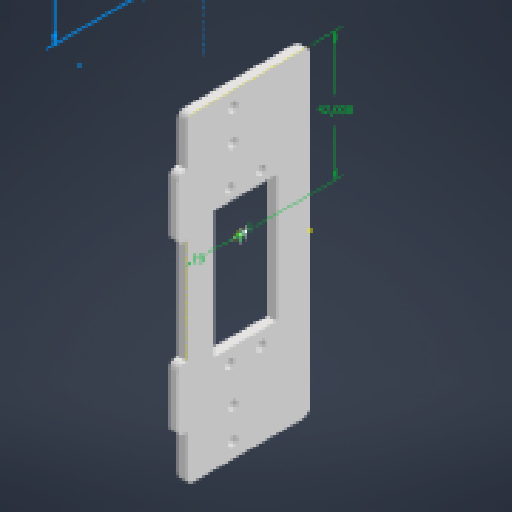
# Autodesk Inventor part: ParedEnsambleMotor
Saved by Autodesk Inventor 2026.2 (Build 302298010, 298A)
## iProperties
Created: 2026-04-28
Part Number: ParedEnsambleMotor
Material: Genérico
Document SubType Name: Modeling
Designer: Jose Carlos
Density: 1 g/cm^3
Appearance: Valor por defecto
Author: Jose Carlos
Autodesk Inventor part; units mm, degrees
ref_plane "YZ Plane" through (0, 0, 0) normal (1, 0, 0) x (0, 1, 0)
ref_plane "XZ Plane" through (0, 0, 0) normal (0, 1, 0) x (-1, 0, 0)
ref_plane "XY Plane" through (0, 0, 0) normal (0, 0, 1) x (1, 0, 0)
sketch "Boceto1" plane through (0, 0, 0) normal (1, 0, 0) x (0, 1, 0)
  line L0 (0, 0) -> (-52.0696, 0)
  line L1 (-52.0696, 0) -> (-52.0696, 40)
  line L2 (-52.0696, 40) -> (0, 40)
  line L3 (0, 40) -> (0, 0)
  line L4 (0, 0) -> (51.9461, 0)
  line L5 (51.9461, 0) -> (51.9461, 40)
  line L6 (51.9461, 40) -> (0, 40)
  line L7 (0, 40) -> (0, 0)
  line L8 (-52.0696, 43) -> (-52.0696, 40) construction
  line L9 (51.9461, 43) -> (51.9461, 40) construction
  line L10 (36.9461, 40) -> (16.9461, 40)
  line L11 (16.9461, 40) -> (16.9461, 43)
  line L12 (16.9461, 43) -> (36.9461, 43)
  line L13 (36.9461, 43) -> (36.9461, 40)
  line L14 (-17.0696, 40) -> (-37.0696, 40)
  line L15 (-37.0696, 40) -> (-37.0696, 43)
  line L16 (-37.0696, 43) -> (-17.0696, 43)
  line L17 (-17.0696, 43) -> (-17.0696, 40)
  point P0 (16.9461, 40)
  dimension "d15" = 40
  dimension "d16" = 20
  dimension "d17" = 3
  dimension "d18" = 15
  dimension "d19" = 3
  dimension "d20" = 20
  dimension "d21" = 15
  constraints: 32 end point, 8 parallel, 5 point on line, 4 horizontal, 4 perpendicular
  measures "d15" distance of L4.end L5.end
  measures "d16" distance of L11.end L12.end
  measures "d17" distance of L10.end L11.end
  measures "d18" distance between parallel lines of L5 L13
  measures "d19" distance of L14.end L15.end
  measures "d20" distance of L15.end L16.end
  measures "d21" distance between parallel lines of L1 L15
extrude "Extrusión1" add sketch "Boceto1" along normal blind 3
sketch "Boceto4" plane through (0, 0, 0) normal (-1, 0, 0) x (0, 0, 1)
  circle A0 centre (25, -37.0696) radius 1.6 construction
  circle A1 centre (25, -47.0696) radius 1.6 construction
  circle A2 centre (25, 36.9461) radius 1.6 construction
  circle A3 centre (25, 46.9461) radius 1.6 construction
  point P0 (0, 0)
hole "Agujero2" at (0, -47.0696, 25) at (0, -37.0696, 25) at (0, 36.9461, 25) at (0, 46.9461, 25) direction (1, 0, 0) diameter 3 end through all
sketch "Boceto5" plane through (3, 0, 0) normal (1, 0, 0) x (0, 0, -1)
  circle A0 centre (-23, 9.9416) radius 1.45 construction
  point P0 (0, 0)
hole "Agujero3" [suppressed]
sketch "ReferenciaEje" plane through (3, 0, 0) normal (1, 0, 0) x (0, 0, -1)
  circle A0 centre (-23, 9.9385) radius 1.65 construction
  line L0 (-40, 16.9461) -> (-40, -17.0696) construction
  line L1 (0, 51.9461) -> (-40, 51.9461) construction
  circle A1 centre (-21, 9.9385) radius 0.5
  point P0 (0, 0)
  dimension "d59" = 19
  dimension "d60" = 42.0076
  dimension "d61" = 1
  constraints: 2 coincident, 1 centre point
  measures "d59" distance from line of L0 point (-21, 9.938)
  measures "d60" distance from line of L1 point (-21, 9.938)
  measures "d61" diameter of A1
sketch "Boceto9" plane through (3, 0, 0) normal (1, 0, 0) x (0, 0, -1)
  circle A0 centre (-15.9, 24.6885) radius 2.25 construction
  circle A1 centre (-26.1, 24.6885) radius 2.25 construction
  circle A2 centre (-15.9, -24.8115) radius 2.25 construction
  circle A3 centre (-26.1, -24.8115) radius 2.25 construction
  point P0 (0, 0)
hole "Agujero4" at (3, 24.6885, 15.9) at (3, 24.6885, 26.1) at (3, -24.8115, 26.1) at (3, -24.8115, 15.9) direction (-1, 0, 0) diameter 3 end through all
sketch "Boceto10" plane through (3, 0, 0) normal (1, 0, 0) x (0, 0, -1)
  line L0 (-11, 19.4385) -> (-11, -19.5615) construction
  line L1 (-30.5, 19.9385) -> (-11.5, 19.9385) construction
  line L2 (-31, -19.6129) -> (-31, 19.4898) construction
  line L3 (-11.4533, -20.0615) -> (-30.5467, -20.0615) construction
  line L4 (-10.8, 20.9385) -> (-31.2, 20.9385)
  line L5 (-31.2, 20.9385) -> (-31.2, -20.2615)
  line L6 (-31.2, -20.2615) -> (-10.8, -20.2615)
  line L7 (-10.8, -20.2615) -> (-10.8, 20.9385)
  point P0 (0, 0)
  point P1 (-11, -0.0615)
  dimension "d53" = 0.2
  dimension "d54" = 0.2
  dimension "d55" = 0.2
  dimension "d56" = 1
  constraints: 8 end point, 2 parallel, 1 horizontal, 1 midpoint, 1 perpendicular
  measures "d53" distance from line of point (-11, -0.062) L7
  measures "d54" distance between parallel lines of L6 L3
  measures "d55" distance between parallel lines of L2 L5
  measures "d56" distance between parallel lines of L1 L4
extrude "Extrusión4" cut sketch "Boceto10" against normal through all
fillet "Empalme1" radius 2 8 edges at (1.5, 51.9461, 0) (1.5, -52.0696, 0) (1.5, -52.0696, 40) (1.5, -37.0696, 43) (1.5, -17.0696, 43) (1.5, 16.9461, 43) (1.5, 36.9461, 43) (1.5, 51.9461, 40)
